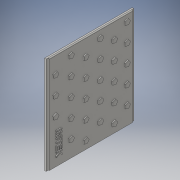
# Autodesk Inventor part: cap
Saved by Autodesk Inventor 2016 (Build 200138000, 138)
## iProperties
Created: 2017-05-23
Part Number: cap
Material: Generic
Document SubType Name: Modeling
Designer: ALIREZA
Density: 1 g/cm^3
Appearance: Default
Author: ALIREZA
Autodesk Inventor part; units mm, degrees
ref_plane "YZ Plane" through (0, 0, 0) normal (1, 0, 0) x (0, 1, 0)
ref_plane "XZ Plane" through (0, 0, 0) normal (0, 1, 0) x (-1, 0, 0)
ref_plane "XY Plane" through (0, 0, 0) normal (0, 0, 1) x (1, 0, 0)
sketch "Sketch1" plane through (0, 0, 0) normal (0, 0, 1) x (1, 0, 0)
  line L0 (22.1383, 85.7995) -> (23.8883, 85.7995)
  line L1 (23.8883, 85.7995) -> (23.8883, 83.3695)
  line L2 (23.8883, 83.3695) -> (24.8883, 83.3695)
  line L3 (24.8883, 83.3695) -> (24.8883, -8.6305)
  line L4 (24.8883, -8.6305) -> (23.8883, -8.6305)
  line L5 (23.8883, -8.6305) -> (23.8883, -11.0605)
  line L6 (23.8883, -11.0605) -> (22.1383, -11.0605)
  line L7 (22.1383, -11.0605) -> (22.1383, 85.7995)
  point P0 (0, 0)
  point P1 (0, 0)
  dimension "d0" = 1.75
  dimension "d1" = 2.43
  dimension "d2" = 1
  dimension "d3" = 92
  dimension "d4" = 1
  dimension "d5" = 2.43
  constraints: 16 end point, 3 horizontal, 3 perpendicular, 2 vertical
  measures "d0" distance of L0.start L0.end
  measures "d1" distance of L0.end L1.end
  measures "d2" distance of L1.end L2.end
  measures "d3" distance of L2.end L3.end
  measures "d4" distance of L3.end L4.end
  measures "d5" distance of L4.end L5.end
extrude "Extrusion1" add sketch "Sketch1" along normal blind 107.5
fillet "Fillet1" radius 1 1 edges at (24.8883, 37.3695, 107.5)
sketch "Sketch2" plane through (24.8883, -8.6305, 0) normal (1, 0, 0) x (0, 0, -1)
  line L0 (-101.4557, 83.1884) -> (-102.7397, 86.6577)
  line L1 (-102.7397, 86.6577) -> (-99.837, 88.951)
  line L2 (-99.837, 88.951) -> (-96.7589, 86.899)
  line L3 (-96.7589, 86.899) -> (-97.7594, 83.3375)
  line L4 (-97.7594, 83.3375) -> (-101.4557, 83.1884)
  line L5 (-99.7101, 85.8067) -> (-3.3014, 85.8067) construction
  line L6 (-81.4557, 83.1884) -> (-82.7397, 86.6577)
  line L7 (-82.7397, 86.6577) -> (-79.837, 88.951)
  line L8 (-79.837, 88.951) -> (-76.7589, 86.899)
  line L9 (-76.7589, 86.899) -> (-77.7594, 83.3375)
  line L10 (-77.7594, 83.3375) -> (-81.4557, 83.1884)
  line L11 (-61.4557, 83.1884) -> (-62.7397, 86.6577)
  line L12 (-62.7397, 86.6577) -> (-59.837, 88.951)
  line L13 (-59.837, 88.951) -> (-56.7589, 86.899)
  line L14 (-56.7589, 86.899) -> (-57.7594, 83.3375)
  line L15 (-57.7594, 83.3375) -> (-61.4557, 83.1884)
  line L16 (-41.4557, 83.1884) -> (-42.7397, 86.6577)
  line L17 (-42.7397, 86.6577) -> (-39.837, 88.951)
  line L18 (-39.837, 88.951) -> (-36.7589, 86.899)
  line L19 (-36.7589, 86.899) -> (-37.7594, 83.3375)
  line L20 (-37.7594, 83.3375) -> (-41.4557, 83.1884)
  line L21 (-21.4557, 83.1884) -> (-22.7397, 86.6577)
  line L22 (-22.7397, 86.6577) -> (-19.837, 88.951)
  line L23 (-19.837, 88.951) -> (-16.7589, 86.899)
  line L24 (-16.7589, 86.899) -> (-17.7594, 83.3375)
  line L25 (-17.7594, 83.3375) -> (-21.4557, 83.1884)
  line L26 (-46.5835, 72.8826) -> (-47.5839, 69.3212)
  line L27 (-49.6615, 74.9346) -> (-46.5835, 72.8826)
  line L28 (-47.5839, 69.3212) -> (-51.2802, 69.1721)
  line L29 (-52.5643, 72.6414) -> (-49.6615, 74.9346)
  line L30 (-31.2802, 69.1721) -> (-32.5643, 72.6414)
  line L31 (-66.5835, 72.8826) -> (-67.5839, 69.3212)
  line L32 (-69.6615, 74.9346) -> (-66.5835, 72.8826)
  line L33 (-67.5839, 69.3212) -> (-71.2802, 69.1721)
  line L34 (-72.5643, 72.6414) -> (-69.6615, 74.9346)
  line L35 (-71.2802, 69.1721) -> (-72.5643, 72.6414)
  line L36 (-51.2802, 69.1721) -> (-52.5643, 72.6414)
  line L37 (-86.5835, 72.8826) -> (-87.5839, 69.3212)
  line L38 (-89.6615, 74.9346) -> (-86.5835, 72.8826)
  line L39 (-87.5839, 69.3212) -> (-91.2802, 69.1721)
  line L40 (-91.2802, 69.1721) -> (-92.5643, 72.6414)
  line L41 (-92.5643, 72.6414) -> (-89.6615, 74.9346)
  line L42 (-6.5835, 72.8826) -> (-7.5839, 69.3212)
  line L43 (-7.5839, 69.3212) -> (-11.2802, 69.1721)
  line L44 (-32.5643, 72.6414) -> (-29.6615, 74.9346)
  line L45 (-27.5839, 69.3212) -> (-31.2802, 69.1721)
  line L46 (-29.6615, 74.9346) -> (-26.5835, 72.8826)
  line L47 (-11.2802, 69.1721) -> (-12.5643, 72.6414)
  line L48 (-12.5643, 72.6414) -> (-9.6615, 74.9346)
  line L49 (-9.6615, 74.9346) -> (-6.5835, 72.8826)
  line L50 (-26.5835, 72.8826) -> (-27.5839, 69.3212)
  line L51 (-55.8659, 57.4867) -> (-56.8663, 53.9252)
  line L52 (-58.9439, 59.5387) -> (-55.8659, 57.4867)
  line L53 (-56.8663, 53.9252) -> (-60.5626, 53.7761)
  line L54 (-61.8466, 57.2454) -> (-58.9439, 59.5387)
  line L55 (-40.5626, 53.7761) -> (-41.8466, 57.2454)
  line L56 (-75.8659, 57.4867) -> (-76.8663, 53.9252)
  line L57 (-78.9439, 59.5387) -> (-75.8659, 57.4867)
  line L58 (-76.8663, 53.9252) -> (-80.5626, 53.7761)
  line L59 (-81.8466, 57.2454) -> (-78.9439, 59.5387)
  line L60 (-80.5626, 53.7761) -> (-81.8466, 57.2454)
  line L61 (-60.5626, 53.7761) -> (-61.8466, 57.2454)
  line L62 (-95.8659, 57.4867) -> (-96.8663, 53.9252)
  line L63 (-98.9439, 59.5387) -> (-95.8659, 57.4867)
  line L64 (-96.8663, 53.9252) -> (-100.5626, 53.7761)
  line L65 (-100.5626, 53.7761) -> (-101.8466, 57.2454)
  line L66 (-101.8466, 57.2454) -> (-98.9439, 59.5387)
  line L67 (-15.8659, 57.4867) -> (-16.8663, 53.9252)
  line L68 (-16.8663, 53.9252) -> (-20.5626, 53.7761)
  line L69 (-41.8466, 57.2454) -> (-38.9439, 59.5387)
  line L70 (-36.8663, 53.9252) -> (-40.5626, 53.7761)
  line L71 (-38.9439, 59.5387) -> (-35.8659, 57.4867)
  line L72 (-20.5626, 53.7761) -> (-21.8466, 57.2454)
  line L73 (-21.8466, 57.2454) -> (-18.9439, 59.5387)
  line L74 (-18.9439, 59.5387) -> (-15.8659, 57.4867)
  line L75 (-35.8659, 57.4867) -> (-36.8663, 53.9252)
  line L76 (-45.9242, 41.2236) -> (-46.9246, 37.6621)
  line L77 (-49.0022, 43.2756) -> (-45.9242, 41.2236)
  line L78 (-46.9246, 37.6621) -> (-50.6209, 37.513)
  line L79 (-51.9049, 40.9824) -> (-49.0022, 43.2756)
  line L80 (-30.6209, 37.513) -> (-31.9049, 40.9824)
  line L81 (-65.9242, 41.2236) -> (-66.9246, 37.6621)
  line L82 (-69.0022, 43.2756) -> (-65.9242, 41.2236)
  line L83 (-66.9246, 37.6621) -> (-70.6209, 37.513)
  line L84 (-71.9049, 40.9824) -> (-69.0022, 43.2756)
  line L85 (-70.6209, 37.513) -> (-71.9049, 40.9824)
  line L86 (-50.6209, 37.513) -> (-51.9049, 40.9824)
  line L87 (-85.9242, 41.2236) -> (-86.9246, 37.6621)
  line L88 (-89.0022, 43.2756) -> (-85.9242, 41.2236)
  line L89 (-86.9246, 37.6621) -> (-90.6209, 37.513)
  line L90 (-90.6209, 37.513) -> (-91.9049, 40.9824)
  line L91 (-91.9049, 40.9824) -> (-89.0022, 43.2756)
  line L92 (-5.9242, 41.2236) -> (-6.9246, 37.6621)
  line L93 (-6.9246, 37.6621) -> (-10.6209, 37.513)
  line L94 (-31.9049, 40.9824) -> (-29.0022, 43.2756)
  line L95 (-26.9246, 37.6621) -> (-30.6209, 37.513)
  line L96 (-29.0022, 43.2756) -> (-25.9242, 41.2236)
  line L97 (-10.6209, 37.513) -> (-11.9049, 40.9824)
  line L98 (-11.9049, 40.9824) -> (-9.0022, 43.2756)
  line L99 (-9.0022, 43.2756) -> (-5.9242, 41.2236)
  line L100 (-25.9242, 41.2236) -> (-26.9246, 37.6621)
  line L101 (-55.4952, 25.0217) -> (-56.4956, 21.4602)
  line L102 (-58.5732, 27.0737) -> (-55.4952, 25.0217)
  line L103 (-56.4956, 21.4602) -> (-60.192, 21.3111)
  line L104 (-61.476, 24.7805) -> (-58.5732, 27.0737)
  line L105 (-40.192, 21.3111) -> (-41.476, 24.7805)
  line L106 (-75.4952, 25.0217) -> (-76.4956, 21.4602)
  line L107 (-78.5732, 27.0737) -> (-75.4952, 25.0217)
  line L108 (-76.4956, 21.4602) -> (-80.192, 21.3111)
  line L109 (-81.476, 24.7805) -> (-78.5732, 27.0737)
  line L110 (-80.192, 21.3111) -> (-81.476, 24.7805)
  line L111 (-60.192, 21.3111) -> (-61.476, 24.7805)
  line L112 (-95.4952, 25.0217) -> (-96.4956, 21.4602)
  line L113 (-98.5732, 27.0737) -> (-95.4952, 25.0217)
  line L114 (-96.4956, 21.4602) -> (-100.192, 21.3111)
  line L115 (-100.192, 21.3111) -> (-101.476, 24.7805)
  line L116 (-101.476, 24.7805) -> (-98.5732, 27.0737)
  line L117 (-15.4952, 25.0217) -> (-16.4956, 21.4602)
  line L118 (-16.4956, 21.4602) -> (-20.192, 21.3111)
  line L119 (-41.476, 24.7805) -> (-38.5732, 27.0737)
  line L120 (-36.4956, 21.4602) -> (-40.192, 21.3111)
  line L121 (-38.5732, 27.0737) -> (-35.4952, 25.0217)
  line L122 (-20.192, 21.3111) -> (-21.476, 24.7805)
  line L123 (-21.476, 24.7805) -> (-18.5732, 27.0737)
  line L124 (-18.5732, 27.0737) -> (-15.4952, 25.0217)
  line L125 (-35.4952, 25.0217) -> (-36.4956, 21.4602)
  line L126 (-90.3467, 4.1864) -> (-91.6308, 7.6557)
  line L127 (-71.6308, 7.6557) -> (-68.728, 9.949)
  line L128 (-68.728, 9.949) -> (-65.65, 7.897)
  line L129 (-65.65, 7.897) -> (-66.6504, 4.3355)
  line L130 (-66.6504, 4.3355) -> (-70.3467, 4.1864)
  line L131 (-70.3467, 4.1864) -> (-71.6308, 7.6557)
  line L132 (-88.728, 9.949) -> (-85.65, 7.897)
  line L133 (-91.6308, 7.6557) -> (-88.728, 9.949)
  line L134 (-85.65, 7.897) -> (-86.6504, 4.3355)
  line L135 (-86.6504, 4.3355) -> (-90.3467, 4.1864)
  line L136 (-51.6308, 7.6557) -> (-48.728, 9.949)
  line L137 (-48.728, 9.949) -> (-45.65, 7.897)
  line L138 (-50.3467, 4.1864) -> (-51.6308, 7.6557)
  line L139 (-46.6504, 4.3355) -> (-50.3467, 4.1864)
  line L140 (-45.65, 7.897) -> (-46.6504, 4.3355)
  line L141 (-35.6152, 13.3324) -> (-3.6818, 13.3324) construction
  line L142 (-3.6818, 13.3324) -> (-3.6818, -0.209) construction
  line L143 (-3.6818, -0.209) -> (-35.6152, -0.209) construction
  line L144 (-35.6152, -0.209) -> (-35.6152, 13.3324) construction
  line L145 (-34.9446, 7.2324) -> (-34.9446, 13.3324)
  line L146 (-34.9446, 13.3324) -> (-33.6878, 13.3324)
  line L147 (-33.6878, 13.3324) -> (-33.6878, 7.2324)
  line L148 (-33.6878, 7.2324) -> (-34.9446, 7.2324)
  line L149 (-32.3764, 7.2324) -> (-32.3764, 13.3324)
  line L150 (-32.3764, 13.3324) -> (-30.5186, 13.3324)
  line L151 (-30.5186, 13.3324) -> (-29.3016, 8.6878)
  line L152 (-29.3016, 8.6878) -> (-28.1045, 13.3324)
  line L153 (-28.1045, 13.3324) -> (-26.2417, 13.3324)
  line L154 (-26.2417, 13.3324) -> (-26.2417, 7.2324)
  line L155 (-26.2417, 7.2324) -> (-27.419, 7.2324)
  line L156 (-27.419, 7.2324) -> (-27.419, 12.1501)
  line L157 (-27.419, 12.1501) -> (-28.6558, 7.2324)
  line L158 (-28.6558, 7.2324) -> (-29.9424, 7.2324)
  line L159 (-29.9424, 7.2324) -> (-31.1992, 12.1501)
  line L160 (-31.1992, 12.1501) -> (-31.1992, 7.2324)
  line L161 (-31.1992, 7.2324) -> (-32.3764, 7.2324)
  line L162 (-23.7133, 7.2324) -> (-23.7133, 12.2445)
  line L163 (-23.7133, 12.2445) -> (-25.5214, 12.2445)
  line L164 (-25.5214, 12.2445) -> (-25.5214, 13.3324)
  line L165 (-25.5214, 13.3324) -> (-20.6583, 13.3324)
  line L166 (-20.6583, 13.3324) -> (-20.6583, 12.2445)
  line L167 (-20.6583, 12.2445) -> (-22.4565, 12.2445)
  line L168 (-22.4565, 12.2445) -> (-22.4565, 7.2324)
  line L169 (-22.4565, 7.2324) -> (-23.7133, 7.2324)
  line L170 (-19.933, 7.2324) -> (-19.933, 13.3324)
  line L171 (-19.933, 13.3324) -> (-15.5021, 13.3324)
  line L172 (-15.5021, 13.3324) -> (-15.5021, 12.2693)
  line L173 (-15.5021, 12.2693) -> (-18.6962, 12.2693)
  line L174 (-18.6962, 12.2693) -> (-18.6962, 10.9679)
  line L175 (-18.6962, 10.9679) -> (-15.7753, 10.9679)
  line L176 (-15.7753, 10.9679) -> (-15.7753, 9.9247)
  line L177 (-15.7753, 9.9247) -> (-18.6962, 9.9247)
  line L178 (-18.6962, 9.9247) -> (-18.6962, 8.36)
  line L179 (-18.6962, 8.36) -> (-15.3531, 8.36)
  line L180 (-15.3531, 8.36) -> (-15.3531, 7.2324)
  line L181 (-15.3531, 7.2324) -> (-19.933, 7.2324)
  line L182 (-14.3944, 7.2324) -> (-14.3944, 13.3324)
  line L183 (-14.3944, 13.3324) -> (-13.1376, 13.3324)
  line L184 (-13.1376, 13.3324) -> (-13.1376, 10.8288)
  line L185 (-13.1376, 10.8288) -> (-10.7532, 13.3324)
  line L186 (-10.7532, 13.3324) -> (-9.1835, 13.3324)
  line L187 (-9.1835, 13.3324) -> (-11.6225, 10.8635)
  line L188 (-11.6225, 10.8635) -> (-8.965, 7.2324)
  line L189 (-8.965, 7.2324) -> (-10.4999, 7.2324)
  line L190 (-10.4999, 7.2324) -> (-12.4869, 10.0241)
  line L191 (-12.4869, 10.0241) -> (-13.1376, 9.3783)
  line L192 (-13.1376, 9.3783) -> (-13.1376, 7.2324)
  line L193 (-13.1376, 7.2324) -> (-14.3944, 7.2324)
  point P0 (0, 8.6305)
  point P1 (-55.8014, 46.9483)
  point P2 (-79.7101, 85.8067)
  point P3 (-59.7101, 85.8067)
  point P4 (-39.7101, 85.8067)
  point P5 (-19.7101, 85.8067)
  point P6 (-49.5347, 71.7904)
  point P7 (-69.5347, 71.7904)
  point P8 (-89.5347, 71.7904)
  point P9 (-29.5347, 71.7904)
  point P10 (-9.5347, 71.7904)
  point P11 (-58.817, 56.3944)
  point P12 (-78.817, 56.3944)
  point P13 (-98.817, 56.3944)
  point P14 (-38.817, 56.3944)
  point P15 (-18.817, 56.3944)
  point P16 (-48.8753, 40.1314)
  point P17 (-68.8753, 40.1314)
  point P18 (-88.8753, 40.1314)
  point P19 (-28.8753, 40.1314)
  point P20 (-8.8753, 40.1314)
  point P21 (-58.4464, 23.9295)
  point P22 (-78.4464, 23.9295)
  point P23 (-98.4464, 23.9295)
  point P24 (-38.4464, 23.9295)
  point P25 (-18.4464, 23.9295)
  point P26 (-68.6012, 6.8047)
  point P27 (-88.6012, 6.8047)
  point P28 (-48.6012, 6.8047)
  point P29 (0, 0)
  dimension "d13" = 20
  dimension "d14" = 20
  dimension "d15" = 20
  dimension "d16" = 20
  dimension "d17" = 20
  dimension "d18" = 20
  constraints: 282 end point, 1 horizontal, 112 other
  measures "d13" distance of L5.start point (-79.71, 85.807)
  measures "d14" distance of point (-89.535, 71.79) point (-69.535, 71.79)
  measures "d15" distance of point (-98.817, 56.394) point (-78.817, 56.394)
  measures "d16" distance of point (-88.875, 40.131) point (-68.875, 40.131)
  measures "d17" distance of point (-98.446, 23.929) point (-78.446, 23.929)
  measures "d18" distance of point (-88.601, 6.805) point (-68.601, 6.805)
extrude "Extrusion2" add sketch "Sketch2" along normal blind 1
body "Solid1"
